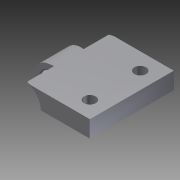
# Autodesk Inventor part: frontissa porta part1
Saved by Autodesk Inventor 2012 SP1 (Build 160190100, 190)
## iProperties
Created: 2015-03-29
Part Number: frontissa porta part1
Material: Default
Document SubType Name: Modeling
Designer: sheina
Density: 1 g/cm^3
Author: sheina
Autodesk Inventor part; units mm, degrees
ref_plane "YZ Plane" through (0, 0, 0) normal (1, 0, 0) x (0, 1, 0)
ref_plane "XZ Plane" through (0, 0, 0) normal (0, 1, 0) x (-1, 0, 0)
ref_plane "XY Plane" through (0, 0, 0) normal (0, 0, 1) x (1, 0, 0)
sketch "Boceto1" plane through (0, 0, 0) normal (0, 0, 1) x (1, 0, 0)
  line L0 (0, 0) -> (20, 0)
  line L1 (20, 0) -> (20, -25)
  line L2 (20, -25) -> (0, -25)
  line L3 (0, -25) -> (0, 0)
  dimension "d0" = 20
  dimension "d1" = 25
  constraints: 8 end point, 2 parallel, 1 horizontal, 1 perpendicular
  measures "d0" distance of L1.end L2.end
  measures "d1" distance of L0.end L1.end
extrude "Extrusión1" add sketch "Boceto1" along normal blind 5
sketch "Boceto4" plane through (0, 0, 5) normal (0, 0, 1) x (1, 0, 0)
  line L0 (20, 0) -> (20, -25) projected
  line L1 (0, 0) -> (20, 0) projected
  circle A0 centre (15, -5) radius 1.75
  circle A1 centre (15, -20) radius 1.75
  point P0 (5, 0)
  dimension "d9" = 3.5
  dimension "d10" = 3.5
  dimension "d11" = 15
  dimension "d12" = 5
  dimension "d13" = 5
  dimension "d14" = 5
  constraints: 2 centre point
  measures "d9" diameter of A0
  measures "d10" diameter of A1
  measures "d11" distance of A1.centre A0.centre
  measures "d12" distance from line of L1 A0.centre
  measures "d13" distance from line of L0 A1.centre
  measures "d14" distance from line of L0 A0.centre
extrude "Extrusión4" cut sketch "Boceto4" against normal blind 25
sketch "Boceto5" plane through (0, 0, 0) normal (0, 1, 0) x (1, 0, 0)
  circle A0 centre (0, 0) radius 5.1
  dimension "d32" = 10.2
  constraints: 1 centre point, 1 coincident
  measures "d32" diameter of A0
extrude "Extrusión5" cut sketch "Boceto5" against normal blind 8.3
sketch "Boceto6" plane through (0, -25, 0) normal (0, -1, 0) x (1, 0, 0)
  circle A0 centre (0, 0) radius 5.1
  dimension "d31" = 10.2
  constraints: 1 centre point, 1 coincident
  measures "d31" diameter of A0
extrude "Extrusión6" cut sketch "Boceto6" against normal blind 8.3
sketch "Boceto7" plane through (0, -16.7, 0) normal (0, -1, 0) x (1, 0, 0)
  line L0 (5.1, 0) -> (0, 0) projected
  arc A0 (5.1, 0) -> (1.005, 5) centre (0, 0) ccw projected
  line L1 (0, 0) -> (0, 5) projected
  circle A1 centre (0, 0) radius 4.9
  dimension "d23" = 9.8
  constraints: 1 centre point, 1 coincident, 1 other
  measures "d23" diameter of A1
extrude "Extrusión7" add sketch "Boceto7" against normal blind 9
sketch "Boceto8" plane through (0, -16.7, 0) normal (0, -1, 0) x (1, 0, 0)
  arc A0 (0, 4.9) -> (4.9, 0) centre (0, 0) ccw projected
  circle A1 centre (0, 0) radius 3
  point P0 (1.005, 5)
  point P1 (5.1, 0)
  dimension "d26" = 6
  constraints: 1 centre point, 1 coincident, 1 other
  measures "d26" diameter of A1
extrude "Extrusión8" cut sketch "Boceto8" against normal blind 9
fillet "Empalme3" radius 0.5 2 edges at (-3, -7.7, 0) (-3, -16.7, 0)
fillet "Empalme4" radius 0.5 2 edges at (3.9456, -25, 3.2315) (3.9456, 0, 3.2315)
